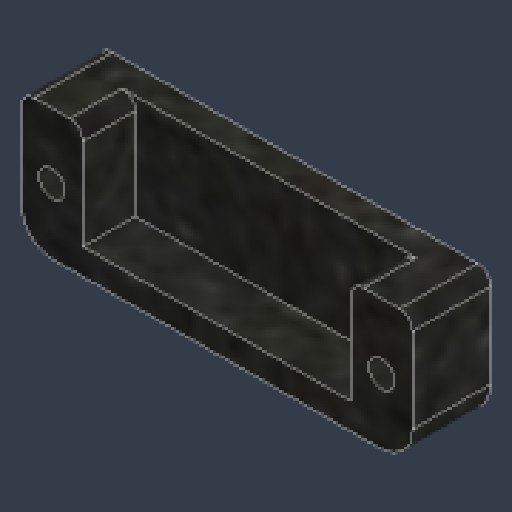
# Autodesk Inventor part: Battery Support
Saved by Autodesk Inventor 2023.4 (Build 274418000, 418)
## iProperties
Created: 2024-07-22
Part Number: Battery Support
Material: Generic
Document SubType Name: Modeling
Designer: JoaoSilva
Density: 1 g/cm^3
Appearance: Smooth - Black
Author: JoaoSilva
Autodesk Inventor part; units mm, degrees
ref_plane "YZ Plane" through (0, 0, 0) normal (1, 0, 0) x (0, 1, 0)
ref_plane "XZ Plane" through (0, 0, 0) normal (0, 1, 0) x (-1, 0, 0)
ref_plane "XY Plane" through (0, 0, 0) normal (0, 0, 1) x (1, 0, 0)
sketch "Sketch1" plane through (0, 0, 0) normal (0, 0, 1) x (1, 0, 0)
  line L0 (-30, 10) -> (30, 10)
  line L1 (30, 10) -> (30, -10)
  line L2 (30, -10) -> (-30, -10)
  line L3 (-30, -10) -> (-30, 10)
  line L4 (-30, 10) -> (30, -10) construction
  line L5 (30, 10) -> (-30, -10) construction
  point P0 (0, 0)
  dimension "d0" = 60
  dimension "d1" = 20
  constraints: 12 end point, 2 midpoint, 2 parallel, 1 horizontal, 1 perpendicular
  measures "d0" distance of L1.end L2.end
  measures "d1" distance of L0.end L1.end
extrude "Extrusion1" add sketch "Sketch1" along normal blind 12
sketch "Sketch2" plane through (0, 0, 12) normal (0, 0, 1) x (1, 0, 0)
  line L0 (-20.5, -6) -> (20.5, -6)
  line L1 (20.5, -6) -> (20.5, 10)
  line L2 (20.5, 10) -> (-20.5, 10)
  line L3 (-20.5, 10) -> (-20.5, -6)
  line L4 (30, 10) -> (-30, 10) projected
  line L5 (-30, -10) -> (30, -10) projected
  point P0 (0, 0)
  point P1 (0, 10)
  dimension "d4" = 41
  dimension "d5" = 4
  constraints: 8 end point, 2 midpoint, 2 parallel, 1 horizontal, 1 perpendicular
  measures "d4" distance between parallel lines of L3 L1
  measures "d5" distance between parallel lines of L5 L0
extrude "Extrusion2" cut sketch "Sketch2" against normal blind 8
sketch "Sketch3" plane through (0, 0, 12) normal (0, 0, 1) x (1, 0, 0)
  line L0 (-25.25, 0) -> (25.25, 0) construction
  line L1 (-30, 10) -> (-30, -10) projected
  line L2 (-20.5, -6) -> (-20.5, 10) projected
  point P0 (0, 0)
  point P1 (0, 0)
  dimension "d8" = 9.5
  dimension "d9" = 4.75
  constraints: 2 end point, 1 coincident, 1 horizontal, 1 midpoint
  measures "d8" distance between parallel lines of L1 L2
  measures "d9" distance from line of L1 L0.start
hole "Hole1" at (-25.25, 0, 12) at (25.25, 0, 12) direction (0, 0, -1) diameter 4 end through all
fillet "Fillet1" radius 2 4 edges at (-30, 10, 6) (-20.5, 10, 8) (20.5, 10, 8) (30, 10, 6)
fillet "Fillet2" radius 5 2 edges at (30, -10, 6) (-30, -10, 6)
equation "\"d9\" = 0.5 * d8"
body "Solid1"
